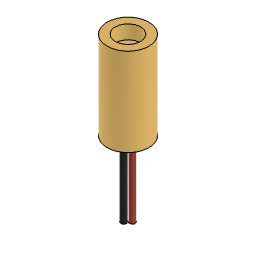
laser module holder (Autodesk Fusion 360 archive; units mm, degrees)
design "Laser Diode"
Autodesk Fusion 360 part; units mm, degrees
sketch "Sketch1" plane through (0, 0, 0) normal (0, 0, 1) x (1, 0, 0)
  circle A0 centre (5, 5) radius 4.75
  dimension "d1" = 9.5
  measures "d1" diameter of A0
extrude "Extrude1" add sketch "Sketch1" along normal blind 20
sketch "Sketch2" plane through (0, 0, 20) normal (0, 0, 1) x (-1, 0, 0)
  circle A0 centre (-5, -5) radius 4.75
  circle A1 centre (-5, -5) radius 2.875
  dimension "d4" = 5.75
  constraint concentric A0 A1
  measures "d4" diameter of A1
extrude "Extrude2" cut sketch "Sketch2" against normal blind 3.15 contours A1
sketch "Sketch3" plane through (0, 0, 16.85) normal (0, 0, 1) x (-1, 0, 0)
  circle A0 centre (-5, -5) radius 2.875
  circle A1 centre (-5, -5) radius 1.6
  dimension "d7" = 3.2
  constraint concentric A0 A1
  measures "d7" diameter of A1
extrude "Extrude3" cut sketch "Sketch3" against normal blind 0.85 contours A1
sketch "Sketch4" plane through (0, 0, 0) normal (0, 0, -1) x (1, 0, 0)
  circle A0 centre (5, -5) radius 4.75
  circle A1 centre (5, -5) radius 1.625
  dimension "d10" = 3.25
  constraint concentric A0 A1
  measures "d10" diameter of A1
extrude "Extrude4" cut sketch "Sketch4" against normal blind 3 contours A1
sketch "Sketch6" plane through (0, 0, 3) normal (0, 0, -1) x (1, 0, 0)
  circle A0 centre (5, -5) radius 1.625
  circle A1 centre (4.5, -4.5) radius 0.65
  circle A2 centre (5.5, -5.5) radius 0.65
  dimension "d13" = 1.3
  dimension "d14" = 1.3
  measures "d13" diameter of A1
  measures "d14" diameter of A2
sketch "Sketch7" plane through (0, 0, 0) normal (0, 0, -1) x (1, 0, 0)
  circle A0 centre (5, -5) radius 1.625
  circle A1 centre (5, -5) radius 4.75
extrude "Extrude5" add sketch "Sketch6" along normal blind 20 contours A1
extrude "Extrude6" add sketch "Sketch6" along normal blind 20 contours A2
